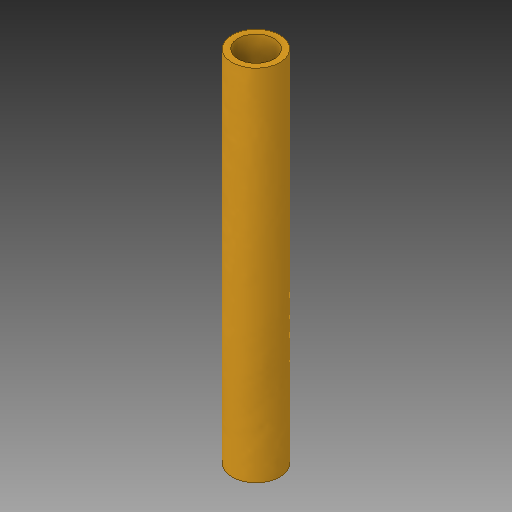
# Autodesk Inventor part: tube_laiton
Saved by Autodesk Inventor 2019 (Build 230136000, 136)
## iProperties
Created: 2017-12-27
Part Number: tube_laiton
Material: Generic
Document SubType Name: Modeling
Designer: franc
Density: 1 g/cm^3
Appearance: Default
Mass: 0.164934 g
Surface Area: 6.7073 cm^2
Volume: 0.164934 cm^3
Author: franc
Autodesk Inventor part; units mm, degrees
ref_plane "YZ Plane" through (0, 0, 0) normal (1, 0, 0) x (0, 1, 0)
ref_plane "XZ Plane" through (0, 0, 0) normal (0, 1, 0) x (-1, 0, 0)
ref_plane "XY Plane" through (0, 0, 0) normal (0, 0, 1) x (1, 0, 0)
sketch "Esquisse1" plane through (0, 0, 0) normal (0, 1, 0) x (-1, 0, 0)
  circle A0 centre (0, 0) radius 1.5
  circle A1 centre (0, 0) radius 2
  dimension "d0" = 4
  dimension "d1" = 3
  constraints: 2 centre point, 2 coincident
  measures "d0" diameter of A1
  measures "d1" diameter of A0
extrude "Extrusion1" add sketch "Esquisse1" along normal blind 30
